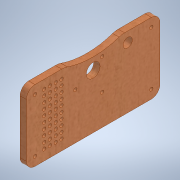
# Autodesk Inventor part: ロボットベースT5.5
Saved by Autodesk Inventor 2020.3 (Build 243373000, 373)
## iProperties
Created: 2020-07-04
Part Number: ロボットベースT5.5
Material: 木材 (クルミ材)
Document SubType Name: Modeling
Designer: totot
Density: 0.55 g/cm^3
Appearance: クルミ材 - ナチュラル つや出し
Mass: 19.4818 g
Surface Area: 175.495 cm^2
Volume: 35.4214 cm^3
Author: totot
Autodesk Inventor part; units mm, degrees
ref_plane "YZ Plane" through (0, 0, 0) normal (1, 0, 0) x (0, 1, 0)
ref_plane "XZ Plane" through (0, 0, 0) normal (0, 1, 0) x (-1, 0, 0)
ref_plane "XY Plane" through (0, 0, 0) normal (0, 0, 1) x (1, 0, 0)
sketch "スケッチ1" plane through (0, 0, 0) normal (1, 0, 0) x (0, 1, 0)
  line L0 (0, 0) -> (-61.5, 0)
  line L1 (-61.5, 0) -> (-61.5, -116)
  line L2 (-61.5, -116) -> (0, -116)
  line L3 (0, -116) -> (0, 0)
  dimension "d0" = 61.5
  dimension "d1" = 116
  constraints: 8 end point, 2 parallel, 1 horizontal, 1 perpendicular
  measures "d0" distance of L2.end L1.end
  measures "d1" distance of L1.end L0.end
extrude "押し出し1" add sketch "スケッチ1" along normal blind 5.5
sketch "スケッチ2" plane through (0, 0, 0) normal (-1, 0, 0) x (0, 0, 1)
  line L0 (-116, -61.5) -> (-116, 0) projected
  line L1 (-116, 0) -> (0, 0) projected
  line L2 (0, -61.5) -> (-116, -61.5) projected
  line L3 (0, 0) -> (0, -61.5) projected
  point P0 (-108.5, -7.5)
  point P1 (-7.5, -7.5)
  point P2 (-7.5, -54)
  point P3 (-108.5, -54)
  dimension "d4" = 7.5
  dimension "d5" = 7.5
  dimension "d6" = 7.5
  dimension "d7" = 7.5
  dimension "d8" = 7.5
  dimension "d9" = 7.5
  dimension "d10" = 7.5
  dimension "d11" = 7.5
  measures "d4" distance from line of point (-108.5, -7.5) L0
  measures "d5" distance from line of point (-108.5, -7.5) L1
  measures "d6" distance from line of L0 point (-108.5, -54)
  measures "d7" distance from line of L2 point (-108.5, -54)
  measures "d8" distance from line of L2 point (-7.5, -54)
  measures "d9" distance from line of L3 point (-7.5, -54)
  measures "d10" distance from line of point (-7.5, -7.5) L1
  measures "d11" distance from line of point (-7.5, -7.5) L3
hole "穴1" at (0, -7.5, -108.5) at (0, -7.5, -7.5) at (0, -54, -7.5) at (0, -54, -108.5) direction (1, 0, 0) diameter 3 end through all
fillet "フィレット1" radius 7.5 4 edges at (2.75, 0, 0) (2.75, -61.5, 0) (2.75, -61.5, -116) (2.75, 0, -116)
sketch "スケッチ3" plane through (0, 0, 0) normal (-1, 0, 0) x (0, 0, 1)
  line L0 (0, -7.5) -> (0, -54) projected
  line L1 (-116, -54) -> (-116, -7.5) projected
  line L2 (-108.5, 0) -> (-7.5, 0) projected
  point P0 (0, 0)
  point P1 (-58, -14.5)
  point P2 (-58, 65.5)
  dimension "d20" = 116
  dimension "d21" = 58
  dimension "d49" = 65.5
  dimension "d50" = 80
  measures "d20" distance between parallel lines of L0 L1
  measures "d21" distance from line of point (-58, -14.5) L1
  measures "d49" distance from line of point (-58, 65.5) L2
  measures "d50" distance of point (-58, -14.5) point (-58, 65.5)
hole "穴2" at (0, -14.5, -58) direction (1, 0, 0) diameter 12 end through all
sketch "スケッチ4" plane through (0, 0, 0) normal (-1, 0, 0) x (0, 0, 1)
  circle A0 centre (-58, -21.5) radius 15.5
  line L0 (-58, -21.5) -> (-42.5, -21.5)
  line L1 (-58, -21.5) -> (-65.75, -34.9234)
  line L2 (-58, -21.5) -> (-42.5, -21.5) construction
  line L3 (-58, -21.5) -> (-65.75, -8.0766)
  circle A1 centre (-58, -14.5) radius 6 projected
  point P0 (0, 0)
  dimension "d31" = 31
  dimension "d32" = 120
  dimension "d33" = 120
  dimension "d51" = 7
  dimension "d52" = 0
  constraints: 8 end point, 3 coincident, 3 point on circle, 2 horizontal, 1 centre point, 1 equal length
  measures "d31" diameter of A0
  measures "d32" angle of L1 L2
  measures "d33" angle of L1 L3
  measures "d51" distance of L0.start A1.centre
  measures "d52" horizontal distance of L0.start A1.centre
hole "穴3" at (0, -21.5, -42.5) at (0, -34.9234, -65.75) at (0, -8.0766, -65.75) direction (1, 0, 0) diameter 3 end through all
sketch "スケッチ5" plane through (0, 0, 0) normal (-1, 0, 0) x (0, 0, 1)
  circle A0 centre (-58, -14.5) radius 6 projected
  circle A1 centre (-58, 65.5) radius 70
  point P0 (0, 0)
  dimension "d42" = 65.5
  dimension "d43" = 58
  dimension "d44" = 58
  dimension "d45" = 140
  constraints: 1 centre point, 1 coincident
  measures "d42" vertical distance of point (-58, 65.5) point (0, 0)
  measures "d43" horizontal distance of point (-58, 65.5) point (0, 0)
  measures "d44" horizontal distance of point (0, 0) A0.centre
  measures "d45" diameter of A1
extrude "押し出し2" cut sketch "スケッチ5" against normal through all contours A1
fillet "フィレット2" radius 15 2 edges at (2.75, 0, -33.3069) (2.75, 0, -82.6931)
sketch "スケッチ6" plane through (0, 0, 0) normal (-1, 0, 0) x (0, 0, 1)
  circle A0 centre (-7.5, -7.5) radius 1.5 projected
  line L0 (-30.7099, 0) -> (-7.5, 0) projected
  line L1 (0, -7.5) -> (0, -54) projected
  point P0 (0, 0)
  point P1 (-15.5, -7.5)
  point P2 (-20.5, -7.5)
  point P3 (-25.5, -7.5)
  point P4 (-15.5, -12.5)
  point P5 (-20.5, -12.5)
  point P6 (-25.5, -12.5)
  point P7 (-15.5, -17.5)
  point P8 (-20.5, -17.5)
  point P9 (-25.5, -17.5)
  point P10 (-15.5, -22.5)
  point P11 (-20.5, -22.5)
  point P12 (-25.5, -22.5)
  point P13 (-15.5, -27.5)
  point P14 (-20.5, -27.5)
  point P15 (-25.5, -27.5)
  point P16 (-15.5, -32.5)
  point P17 (-20.5, -32.5)
  point P18 (-25.5, -32.5)
  point P19 (-15.5, -37.5)
  point P20 (-20.5, -37.5)
  point P21 (-25.5, -37.5)
  point P22 (-15.5, -42.5)
  point P23 (-20.5, -42.5)
  point P24 (-25.5, -42.5)
  point P25 (-15.5, -47.5)
  point P26 (-20.5, -47.5)
  point P27 (-25.5, -47.5)
  point P28 (-15.5, -52.5)
  point P29 (-20.5, -52.5)
  point P30 (-25.5, -52.5)
  point P31 (-30.5, -7.5)
  point P32 (-30.5, -12.5)
  point P33 (-30.5, -17.5)
  point P34 (-30.5, -22.5)
  point P35 (-30.5, -27.5)
  point P36 (-30.5, -32.5)
  point P37 (-30.5, -37.5)
  point P38 (-30.5, -42.5)
  point P39 (-30.5, -47.5)
  point P40 (-30.5, -52.5)
  dimension "d53" = 8
  dimension "d54" = 7.5
  dimension "d64" = 5
  dimension "d69" = 15.5
  dimension "d72" = 5
  dimension "d79" = 5
  constraints: 2 horizontal, 1 vertical, 39 other
  measures "d53" distance of point (-15.5, -7.5) A0.centre
  measures "d54" distance from line of L0 point (-15.5, -7.5)
  measures "d64" distance of point (-15.5, -7.5) point (-20.5, -7.5)
  measures "d69" distance from line of point (-15.5, -7.5) L1
  measures "d72" distance of point (-15.5, -7.5) point (-15.5, -12.5)
  measures "d79" distance of point (-25.5, -7.5) point (-30.5, -7.5)
hole "穴4" at (0, -7.5, -15.5) at (0, -7.5, -20.5) at (0, -7.5, -25.5) at (0, -12.5, -15.5) at (0, -12.5, -20.5) at (0, -12.5, -25.5) at (0, -17.5, -15.5) at (0, -17.5, -20.5) at (0, -17.5, -25.5) at (0, -22.5, -15.5) at (0, -22.5, -20.5) at (0, -22.5, -25.5) at (0, -27.5, -15.5) at (0, -27.5, -20.5) at (0, -27.5, -25.5) at (0, -32.5, -15.5) at (0, -32.5, -20.5) at (0, -32.5, -25.5) at (0, -37.5, -15.5) at (0, -37.5, -20.5) at (0, -37.5, -25.5) at (0, -42.5, -15.5) at (0, -42.5, -20.5) at (0, -42.5, -25.5) at (0, -47.5, -15.5) at (0, -47.5, -20.5) at (0, -47.5, -25.5) at (0, -52.5, -15.5) at (0, -52.5, -20.5) at (0, -52.5, -25.5) at (0, -7.5, -30.5) at (0, -12.5, -30.5) at (0, -17.5, -30.5) at (0, -22.5, -30.5) at (0, -27.5, -30.5) at (0, -32.5, -30.5) at (0, -37.5, -30.5) at (0, -42.5, -30.5) at (0, -47.5, -30.5) at (0, -52.5, -30.5) direction (1, 0, 0) diameter 3 end through all
sketch "スケッチ7" plane through (0, 0, 0) normal (-1, 0, 0) x (0, 0, 1)
  circle A0 centre (-87.9685, -8.6747) radius 4
  circle A1 centre (-58, 65.5) radius 80
  line L0 (0, -7.5) -> (0, -54) projected
  line L1 (-116, -54) -> (-116, -7.5) projected
  circle A2 centre (-58, -14.5) radius 6 projected
  line L2 (-58, 65.5) -> (-87.9685, -8.6747)
  line L3 (-58, 65.5) -> (-58, -14.5)
  point P0 (0, 0)
  dimension "d94" = 160
  dimension "d91" = 8
  dimension "d95" = 116
  dimension "d96" = 58
  dimension "d97" = 80
  dimension "d98" = 22
  constraints: 4 end point, 1 centre point, 1 coincident, 3 other
  measures "d91" diameter of A0
  measures "d95" distance between parallel lines of L0 L1
  measures "d96" distance from line of L1 L2.start
  measures "d97" distance of L3.end L2.start
  measures "d98" angle of L3 L2
extrude "押し出し3" cut sketch "スケッチ7" against normal through all contours A0 A1 L2 | L2 A1 A0 | A0 A1
equation "\"d5\" = d4"
equation "\"d6\" = d5"
equation "\"d7\" = d6"
equation "\"d8\" = d6"
equation "\"d9\" = d8"
equation "\"d10\" = d8"
equation "\"d11\" = d10"
equation "\"d21\" = 0.5 * d20"
equation "\"d43\" = d44"
equation "\"d96\" = 0.5 * d95"
equation "\"d97\" = 0.5 * d94"
